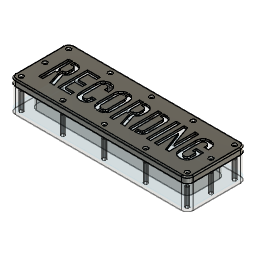
RECORDING sign (Autodesk Fusion 360 design; units mm, degrees)
Autodesk Fusion 360 part; units mm, degrees
note: some values were not read from the file. Set by a fixed rule: which sketch regions a step uses.
(part 1 of 2)
sketch "Esquisse1" plane through (0, 0, 0) normal (0, 0, 1) x (1, 0, 0)
  line L0 (0, 0) -> (300, 0)
  line L1 (300, 0) -> (300, -100)
  line L2 (300, -100) -> (0, -100)
  line L3 (0, -100) -> (0, 0)
  circle A0 centre (10, -10) radius 1.7
  circle A1 centre (290, -10) radius 1.7
  circle A2 centre (10, -90) radius 1.7
  circle A3 centre (290, -90) radius 1.7
  circle A4 centre (150, -10) radius 1.7
  circle A5 centre (150, -90) radius 1.7
  circle A6 centre (80, -10) radius 1.7
  circle A7 centre (80, -90) radius 1.7
  circle A8 centre (10, -50) radius 1.7
  circle A9 centre (290, -50) radius 1.7
  circle A10 centre (220, -10) radius 1.7
  circle A11 centre (220, -90) radius 1.7
  line L4 (27.716637, -53.851447) -> (27.716637, -47.661624)
  line L5 (27.716637, -47.661624) -> (36.932595, -47.661624)
  spline S0 degree 2 poles (36.932595, -47.661624) (39.580462, -47.661624) (41.041949, -46.200137) knots 0 0 0 1 1 1
  spline S1 degree 2 poles (41.041949, -46.200137) (42.503434, -44.73865) (42.503434, -42.125173) knots 0 0 0 1 1 1
  line L6 (42.503434, -42.125173) -> (42.503434, -37.035763)
  spline S2 degree 2 poles (42.503434, -37.035763) (42.503434, -34.250345) (41.041949, -32.702889) knots 0 0 0 1 1 1
  spline S3 degree 2 poles (41.041949, -32.702889) (39.580462, -31.155434) (36.932595, -31.155434) knots 0 0 0 1 1 1
  line L7 (36.932595, -31.155434) -> (27.716637, -31.155434)
  line L8 (27.716637, -31.155434) -> (27.716637, -24.965611)
  line L9 (27.716637, -24.965611) -> (36.348, -24.965611)
  spline S4 degree 2 poles (36.348, -24.965611) (40.371383, -24.965611) (43.208385, -26.289544) knots 0 0 0 1 1 1
  spline S5 degree 2 poles (43.208385, -26.289544) (46.045387, -27.613478) (47.541261, -30.158181) knots 0 0 0 1 1 1
  spline S6 degree 2 poles (47.541261, -30.158181) (49.037133, -32.702889) (49.037133, -36.313617) knots 0 0 0 1 1 1
  line L10 (49.037133, -36.313617) -> (49.037133, -42.159562)
  spline S7 degree 2 poles (49.037133, -42.159562) (49.037133, -45.873451) (47.541261, -48.486934) knots 0 0 0 1 1 1
  spline S8 degree 2 poles (47.541261, -48.486934) (46.045387, -51.100411) (43.208385, -52.475924) knots 0 0 0 1 1 1
  spline S9 degree 2 poles (43.208385, -52.475924) (40.371383, -53.851447) (36.348, -53.851447) knots 0 0 0 1 1 1
  line L11 (36.348, -53.851447) -> (27.716637, -53.851447)
  line L12 (24.656115, -75) -> (24.656115, -24.965611)
  line L13 (24.656115, -24.965611) -> (31.189815, -24.965611)
  line L14 (31.189815, -24.965611) -> (31.189815, -75)
  line L15 (31.189815, -75) -> (24.656115, -75)
  line L16 (43.294354, -75) -> (36.313612, -52.303987)
  line L17 (36.313612, -52.303987) -> (42.469044, -50.722146)
  line L18 (42.469044, -50.722146) -> (50.447038, -75)
  line L19 (50.447038, -75) -> (43.294354, -75)
  line L20 (56.464918, -75) -> (56.464918, -25)
  line L21 (56.464918, -25) -> (62.998617, -25)
  line L22 (62.998617, -25) -> (62.998617, -75)
  line L23 (62.998617, -75) -> (56.464918, -75)
  line L24 (59.869321, -75) -> (59.869321, -68.810177)
  line L25 (59.869321, -68.810177) -> (77.922962, -68.810177)
  line L26 (77.922962, -68.810177) -> (77.922962, -75)
  line L27 (77.922962, -75) -> (59.869321, -75)
  line L28 (59.869321, -53.26685) -> (59.869321, -47.077031)
  line L29 (59.869321, -47.077031) -> (76.203568, -47.077031)
  line L30 (76.203568, -47.077031) -> (76.203568, -53.26685)
  line L31 (76.203568, -53.26685) -> (59.869321, -53.26685)
  line L32 (59.869321, -31.189818) -> (59.869321, -25)
  line L33 (59.869321, -25) -> (77.922962, -25)
  line L34 (77.922962, -25) -> (77.922962, -31.189818)
  line L35 (77.922962, -31.189818) -> (59.869321, -31.189818)
  spline S10 degree 2 poles (94.704254, -75.515819) (91.02475, -75.515819) (88.428467, -74.002752) knots 0 0 0 1 1 1
  spline S11 degree 2 poles (88.428467, -74.002752) (85.832179, -72.489686) (84.456666, -69.635487) knots 0 0 0 1 1 1
  spline S12 degree 2 poles (84.456666, -69.635487) (83.081148, -66.781292) (83.081148, -62.723522) knots 0 0 0 1 1 1
  line L36 (83.081148, -62.723522) -> (83.081148, -37.310865)
  spline S13 degree 2 poles (83.081148, -37.310865) (83.081148, -33.218708) (84.456666, -30.364509) knots 0 0 0 1 1 1
  spline S14 degree 2 poles (84.456666, -30.364509) (85.832179, -27.510314) (88.428467, -25.997248) knots 0 0 0 1 1 1
  spline S15 degree 2 poles (88.428467, -25.997248) (91.02475, -24.484181) (94.704254, -24.484181) knots 0 0 0 1 1 1
  spline S16 degree 2 poles (94.704254, -24.484181) (98.418148, -24.484181) (101.014431, -25.997248) knots 0 0 0 1 1 1
  spline S17 degree 2 poles (101.014431, -25.997248) (103.610723, -27.510314) (104.969042, -30.364509) knots 0 0 0 1 1 1
  spline S18 degree 2 poles (104.969042, -30.364509) (106.32736, -33.218708) (106.32736, -37.276478) knots 0 0 0 1 1 1
  line L37 (106.32736, -37.276478) -> (106.32736, -39.408526)
  line L38 (106.32736, -39.408526) -> (99.724891, -39.408526)
  line L39 (99.724891, -39.408526) -> (99.724891, -37.276478)
  spline S19 degree 2 poles (99.724891, -37.276478) (99.724891, -35.213203) (99.140289, -33.786106) knots 0 0 0 1 1 1
  spline S20 degree 2 poles (99.140289, -33.786106) (98.555706, -32.359009) (97.438095, -31.602473) knots 0 0 0 1 1 1
  spline S21 degree 2 poles (97.438095, -31.602473) (96.320489, -30.845942) (94.704254, -30.845942) knots 0 0 0 1 1 1
  spline S22 degree 2 poles (94.704254, -30.845942) (92.331493, -30.845942) (91.00756, -32.530947) knots 0 0 0 1 1 1
  spline S23 degree 2 poles (91.00756, -32.530947) (89.683626, -34.215956) (89.683626, -37.310865) knots 0 0 0 1 1 1
  line L40 (89.683626, -37.310865) -> (89.683626, -62.723522)
  spline S24 degree 2 poles (89.683626, -62.723522) (89.683626, -65.784044) (91.00756, -67.469049) knots 0 0 0 1 1 1
  spline S25 degree 2 poles (91.00756, -67.469049) (92.331493, -69.154058) (94.704254, -69.154058) knots 0 0 0 1 1 1
  spline S26 degree 2 poles (94.704254, -69.154058) (97.111404, -69.154058) (98.418148, -67.469049) knots 0 0 0 1 1 1
  spline S27 degree 2 poles (98.418148, -67.469049) (99.724891, -65.784044) (99.724891, -62.723522) knots 0 0 0 1 1 1
  line L41 (99.724891, -62.723522) -> (99.724891, -60.591474)
  line L42 (99.724891, -60.591474) -> (106.32736, -60.591474)
  line L43 (106.32736, -60.591474) -> (106.32736, -62.723522)
  spline S28 degree 2 poles (106.32736, -62.723522) (106.32736, -66.781292) (104.969042, -69.635487) knots 0 0 0 1 1 1
  spline S29 degree 2 poles (104.969042, -69.635487) (103.610723, -72.489686) (101.014431, -74.002752) knots 0 0 0 1 1 1
  spline S30 degree 2 poles (101.014431, -74.002752) (98.418148, -75.515819) (94.704254, -75.515819) knots 0 0 0 1 1 1
  spline S31 degree 2 poles (124.931219, -75.515819) (121.010998, -75.515819) (118.225572, -74.037137) knots 0 0 0 1 1 1
  spline S32 degree 2 poles (118.225572, -74.037137) (115.440157, -72.55846) (113.97867, -69.755845) knots 0 0 0 1 1 1
  spline S33 degree 2 poles (113.97867, -69.755845) (112.517183, -66.953235) (112.517183, -62.964234) knots 0 0 0 1 1 1
  line L44 (112.517183, -62.964234) -> (112.517183, -37.035763)
  spline S34 degree 2 poles (112.517183, -37.035763) (112.517183, -33.012381) (113.97867, -30.209765) knots 0 0 0 1 1 1
  spline S35 degree 2 poles (113.97867, -30.209765) (115.440157, -27.40715) (118.225572, -25.945668) knots 0 0 0 1 1 1
  spline S36 degree 2 poles (118.225572, -25.945668) (121.010998, -24.484181) (124.931219, -24.484181) knots 0 0 0 1 1 1
  spline S37 degree 2 poles (124.931219, -24.484181) (128.88582, -24.484181) (131.654051, -25.945668) knots 0 0 0 1 1 1
  spline S38 degree 2 poles (131.654051, -25.945668) (134.422272, -27.40715) (135.883758, -30.209765) knots 0 0 0 1 1 1
  spline S39 degree 2 poles (135.883758, -30.209765) (137.345245, -33.012381) (137.345245, -37.035763) knots 0 0 0 1 1 1
  line L45 (137.345245, -37.035763) -> (137.345245, -62.964234)
  spline S40 degree 2 poles (137.345245, -62.964234) (137.345245, -66.953235) (135.883758, -69.755845) knots 0 0 0 1 1 1
  spline S41 degree 2 poles (135.883758, -69.755845) (134.422272, -72.55846) (131.654051, -74.037137) knots 0 0 0 1 1 1
  spline S42 degree 2 poles (131.654051, -74.037137) (128.88582, -75.515819) (124.931219, -75.515819) knots 0 0 0 1 1 1
  spline S43 degree 2 poles (124.931219, -69.154058) (127.716635, -69.154058) (129.264086, -67.572217) knots 0 0 0 1 1 1
  spline S44 degree 2 poles (129.264086, -67.572217) (130.811546, -65.990372) (130.811546, -63.170562) knots 0 0 0 1 1 1
  line L46 (130.811546, -63.170562) -> (130.811546, -36.829436)
  spline S45 degree 2 poles (130.811546, -36.829436) (130.811546, -33.975239) (129.264086, -32.410588) knots 0 0 0 1 1 1
  spline S46 degree 2 poles (129.264086, -32.410588) (127.716635, -30.845942) (124.931219, -30.845942) knots 0 0 0 1 1 1
  spline S47 degree 2 poles (124.931219, -30.845942) (122.111404, -30.845942) (120.581148, -32.410588) knots 0 0 0 1 1 1
  spline S48 degree 2 poles (120.581148, -32.410588) (119.050882, -33.975239) (119.050882, -36.829436) knots 0 0 0 1 1 1
  line L47 (119.050882, -36.829436) -> (119.050882, -63.170562)
  spline S49 degree 2 poles (119.050882, -63.170562) (119.050882, -65.990372) (120.581148, -67.572217) knots 0 0 0 1 1 1
  spline S50 degree 2 poles (120.581148, -67.572217) (122.111404, -69.154058) (124.931219, -69.154058) knots 0 0 0 1 1 1
  line L48 (147.283352, -53.851447) -> (147.283352, -47.661624)
  line L49 (147.283352, -47.661624) -> (156.499307, -47.661624)
  spline S51 degree 2 poles (156.499307, -47.661624) (159.147175, -47.661624) (160.608661, -46.200137) knots 0 0 0 1 1 1
  spline S52 degree 2 poles (160.608661, -46.200137) (162.070148, -44.73865) (162.070148, -42.125173) knots 0 0 0 1 1 1
  line L50 (162.070148, -42.125173) -> (162.070148, -37.035763)
  spline S53 degree 2 poles (162.070148, -37.035763) (162.070148, -34.250345) (160.608661, -32.702889) knots 0 0 0 1 1 1
  spline S54 degree 2 poles (160.608661, -32.702889) (159.147175, -31.155434) (156.499307, -31.155434) knots 0 0 0 1 1 1
  line L51 (156.499307, -31.155434) -> (147.283352, -31.155434)
  line L52 (147.283352, -31.155434) -> (147.283352, -24.965611)
  line L53 (147.283352, -24.965611) -> (155.914715, -24.965611)
  spline S55 degree 2 poles (155.914715, -24.965611) (159.938095, -24.965611) (162.775095, -26.289544) knots 0 0 0 1 1 1
  spline S56 degree 2 poles (162.775095, -26.289544) (165.612104, -27.613478) (167.107981, -30.158181) knots 0 0 0 1 1 1
  spline S57 degree 2 poles (167.107981, -30.158181) (168.603847, -32.702889) (168.603847, -36.313617) knots 0 0 0 1 1 1
  line L54 (168.603847, -36.313617) -> (168.603847, -42.159562)
  spline S58 degree 2 poles (168.603847, -42.159562) (168.603847, -45.873451) (167.107981, -48.486934) knots 0 0 0 1 1 1
  spline S59 degree 2 poles (167.107981, -48.486934) (165.612104, -51.100411) (162.775095, -52.475924) knots 0 0 0 1 1 1
  spline S60 degree 2 poles (162.775095, -52.475924) (159.938095, -53.851447) (155.914715, -53.851447) knots 0 0 0 1 1 1
  line L55 (155.914715, -53.851447) -> (147.283352, -53.851447)
  line L56 (144.22283, -75) -> (144.22283, -24.965611)
  line L57 (144.22283, -24.965611) -> (150.756529, -24.965611)
  line L58 (150.756529, -24.965611) -> (150.756529, -75)
  line L59 (150.756529, -75) -> (144.22283, -75)
  line L60 (162.861069, -75) -> (155.880325, -52.303987)
  line L61 (155.880325, -52.303987) -> (162.035759, -50.722146)
  line L62 (162.035759, -50.722146) -> (170.01375, -75)
  line L63 (170.01375, -75) -> (162.861069, -75)
  line L64 (180.192573, -75) -> (180.192573, -68.810177)
  line L65 (180.192573, -68.810177) -> (189.305351, -68.810177)
  spline S61 degree 2 poles (189.305351, -68.810177) (191.093529, -68.810177) (192.056396, -67.72696) knots 0 0 0 1 1 1
  spline S62 degree 2 poles (192.056396, -67.72696) (193.019264, -66.643739) (193.019264, -64.718018) knots 0 0 0 1 1 1
  line L66 (193.019264, -64.718018) -> (193.019264, -35.28198)
  spline S63 degree 2 poles (193.019264, -35.28198) (193.019264, -33.356256) (192.056396, -32.27304) knots 0 0 0 1 1 1
  spline S64 degree 2 poles (192.056396, -32.27304) (191.093529, -31.189818) (189.305351, -31.189818) knots 0 0 0 1 1 1
  line L67 (189.305351, -31.189818) -> (180.192573, -31.189818)
  line L68 (180.192573, -31.189818) -> (180.192573, -25)
  line L69 (180.192573, -25) -> (189.099052, -25)
  spline S65 degree 2 poles (189.099052, -25) (194.119652, -25) (196.836326, -27.716641) knots 0 0 0 1 1 1
  spline S66 degree 2 poles (196.836326, -27.716641) (199.552963, -30.433288) (199.552963, -35.45392) knots 0 0 0 1 1 1
  line L70 (199.552963, -35.45392) -> (199.552963, -64.54608)
  spline S67 degree 2 poles (199.552963, -64.54608) (199.552963, -67.847319) (198.314979, -70.202889) knots 0 0 0 1 1 1
  spline S68 degree 2 poles (198.314979, -70.202889) (197.077034, -72.55846) (194.738663, -73.77923) knots 0 0 0 1 1 1
  spline S69 degree 2 poles (194.738663, -73.77923) (192.400291, -75) (189.064644, -75) knots 0 0 0 1 1 1
  line L71 (189.064644, -75) -> (180.192573, -75)
  line L72 (176.031635, -75) -> (176.031635, -25)
  line L73 (176.031635, -25) -> (182.565353, -25)
  line L74 (182.565353, -25) -> (182.565353, -75)
  line L75 (182.565353, -75) -> (176.031635, -75)
  line L76 (212.895477, -25) -> (212.895477, -75)
  line L77 (212.895477, -75) -> (206.361778, -75)
  line L78 (206.361778, -75) -> (206.361778, -25)
  line L79 (206.361778, -25) -> (212.895477, -25)
  line L80 (219.704254, -74.965611) -> (219.704254, -24.999995)
  line L81 (219.704254, -24.999995) -> (225.412643, -24.999995)
  line L82 (225.412643, -24.999995) -> (239.099052, -63.3425)
  line L83 (239.099052, -63.3425) -> (238.032997, -64.236588)
  line L84 (238.032997, -64.236588) -> (238.032997, -24.999995)
  line L85 (238.032997, -24.999995) -> (244.25721, -24.999995)
  line L86 (244.25721, -24.999995) -> (244.25721, -74.965611)
  line L87 (244.25721, -74.965611) -> (238.480041, -74.965611)
  line L88 (238.480041, -74.965611) -> (224.862449, -37.826684)
  line L89 (224.862449, -37.826684) -> (225.928467, -36.932597)
  line L90 (225.928467, -36.932597) -> (225.928467, -74.965611)
  line L91 (225.928467, -74.965611) -> (219.704254, -74.965611)
  line L92 (263.170593, -48.074279) -> (275.343902, -48.074279)
  line L93 (275.343902, -48.074279) -> (275.343902, -62.689133)
  spline S70 degree 2 poles (275.343902, -62.689133) (275.343902, -66.746907) (273.93399, -69.618297) knots 0 0 0 1 1 1
  spline S71 degree 2 poles (273.93399, -69.618297) (272.524078, -72.489686) (269.841812, -74.002752) knots 0 0 0 1 1 1
  spline S72 degree 2 poles (269.841812, -74.002752) (267.159584, -75.515819) (263.342521, -75.515819) knots 0 0 0 1 1 1
  spline S73 degree 2 poles (263.342521, -75.515819) (259.45668, -75.515819) (256.722839, -74.088721) knots 0 0 0 1 1 1
  spline S74 degree 2 poles (256.722839, -74.088721) (253.988998, -72.661624) (252.56192, -69.962173) knots 0 0 0 1 1 1
  spline S75 degree 2 poles (252.56192, -69.962173) (251.134804, -67.262721) (251.134804, -63.411279) knots 0 0 0 1 1 1
  line L94 (251.134804, -63.411279) -> (251.134804, -37.310865)
  spline S76 degree 2 poles (251.134804, -37.310865) (251.134804, -33.218708) (252.544716, -30.364509) knots 0 0 0 1 1 1
  spline S77 degree 2 poles (252.544716, -30.364509) (253.954628, -27.510314) (256.636894, -25.997248) knots 0 0 0 1 1 1
  spline S78 degree 2 poles (256.636894, -25.997248) (259.319122, -24.484181) (263.136185, -24.484181) knots 0 0 0 1 1 1
  spline S79 degree 2 poles (263.136185, -24.484181) (266.884468, -24.484181) (269.515159, -25.945668) knots 0 0 0 1 1 1
  spline S80 degree 2 poles (269.515159, -25.945668) (272.145813, -27.40715) (273.538521, -30.192571) knots 0 0 0 1 1 1
  spline S81 degree 2 poles (273.538521, -30.192571) (274.931228, -32.977991) (274.931228, -36.9326) knots 0 0 0 1 1 1
  line L95 (274.931228, -36.9326) -> (274.931228, -39.408526)
  line L96 (274.931228, -39.408526) -> (267.984894, -39.408526)
  line L97 (267.984894, -39.408526) -> (267.984894, -36.9326)
  spline S82 degree 2 poles (267.984894, -36.9326) (267.984894, -34.009628) (266.729706, -32.427783) knots 0 0 0 1 1 1
  spline S83 degree 2 poles (266.729706, -32.427783) (265.474556, -30.845942) (263.136185, -30.845942) knots 0 0 0 1 1 1
  spline S84 degree 2 poles (263.136185, -30.845942) (260.522697, -30.845942) (259.095619, -32.530947) knots 0 0 0 1 1 1
  spline S85 degree 2 poles (259.095619, -32.530947) (257.668503, -34.215956) (257.668503, -37.310865) knots 0 0 0 1 1 1
  line L98 (257.668503, -37.310865) -> (257.668503, -63.411279)
  spline S86 degree 2 poles (257.668503, -63.411279) (257.668503, -66.127925) (259.147194, -67.640991) knots 0 0 0 1 1 1
  spline S87 degree 2 poles (259.147194, -67.640991) (260.625885, -69.154058) (263.342521, -69.154058) knots 0 0 0 1 1 1
  spline S88 degree 2 poles (263.342521, -69.154058) (265.9216, -69.154058) (267.365883, -67.486243) knots 0 0 0 1 1 1
  spline S89 degree 2 poles (267.365883, -67.486243) (268.810203, -65.818434) (268.810203, -62.792296) knots 0 0 0 1 1 1
  line L99 (268.810203, -62.792296) -> (268.810203, -54.264102)
  line L100 (268.810203, -54.264102) -> (263.170593, -54.264102)
  line L101 (263.170593, -54.264102) -> (263.170593, -48.074279)
  line L102 (31.189815, -24.965611) -> (34.189815, -24.965611)
  line L103 (34.189815, -24.965611) -> (34.189815, -31.155434)
  line L104 (34.189815, -31.155434) -> (31.189815, -31.155434)
  line L105 (31.189815, -31.155434) -> (31.189815, -24.965611)
  line L106 (36.799999, -53.999999) -> (33.799999, -53.999999)
  line L107 (33.799999, -53.999999) -> (33.799999, -47.661624)
  line L108 (33.799999, -47.661624) -> (36.799999, -47.661624)
  line L109 (36.799999, -47.661624) -> (36.799999, -53.999999)
  line L110 (123.500002, -31.5) -> (126.500002, -31.5)
  line L111 (126.500002, -31.5) -> (126.500002, -24)
  line L112 (126.500002, -24) -> (123.500002, -24)
  line L113 (123.500002, -24) -> (123.500002, -31.5)
  line L114 (123.500002, -68.500001) -> (126.500002, -68.500001)
  line L115 (126.500002, -68.500001) -> (126.500002, -76.000001)
  line L116 (126.500002, -76.000001) -> (123.500002, -76.000001)
  line L117 (123.500002, -76.000001) -> (123.500002, -68.500001)
  line L118 (150.756529, -24.965611) -> (153.756529, -24.965611)
  line L119 (153.756529, -24.965611) -> (153.756529, -31.155434)
  line L120 (153.756529, -31.155434) -> (150.756529, -31.155434)
  line L121 (150.756529, -31.155434) -> (150.756529, -24.965611)
  line L122 (156.349997, -53.899999) -> (153.349997, -53.899999)
  line L123 (153.349997, -53.899999) -> (153.349997, -47.661624)
  line L124 (153.349997, -47.661624) -> (156.349997, -47.661624)
  line L125 (156.349997, -47.661624) -> (156.349997, -53.899999)
  line L126 (182.565353, -25) -> (185.565353, -25)
  line L127 (185.565353, -25) -> (185.565353, -31.189818)
  line L128 (185.565353, -31.189818) -> (182.565353, -31.189818)
  line L129 (182.565353, -31.189818) -> (182.565353, -25)
  line L130 (182.565353, -68.810177) -> (185.565353, -68.810177)
  line L131 (185.565353, -68.810177) -> (185.565353, -75.000001)
  line L132 (185.565353, -75.000001) -> (182.565353, -75.000001)
  line L133 (182.565353, -75.000001) -> (182.565353, -68.810177)
  dimension "d35" = 300
  dimension "d36" = 100
  dimension "d37" = 3.4
  dimension "d38" = 3.4
  dimension "d39" = 3.4
  dimension "d40" = 3.4
  dimension "d41" = 3.4
  dimension "d42" = 3.4
  dimension "d43" = 3.4
  dimension "d44" = 3.4
  dimension "d45" = 3.4
  dimension "d46" = 3.4
  dimension "d47" = 3.4
  dimension "d48" = 3.4
  dimension "d50" = 3
  dimension "d51" = 3
  dimension "d52" = 3
  dimension "d53" = 3
  dimension "d54" = 3
  dimension "d55" = 3
  constraint horizontal L0
  constraint vertical L1
  constraint horizontal L2
  constraint vertical L3
  constraint coincident L0.start L3.end
  constraint horizontal L102
  constraint vertical L103
  constraint horizontal L104
  constraint vertical L105
  constraint horizontal L106
  constraint vertical L107
  constraint horizontal L108
  constraint vertical L109
  constraint horizontal L110
  constraint vertical L111
  constraint horizontal L112
  constraint vertical L113
  constraint horizontal L114
  constraint vertical L115
  constraint horizontal L116
  constraint vertical L117
  constraint horizontal L118
  constraint vertical L119
  constraint horizontal L120
  constraint vertical L121
  constraint horizontal L122
  constraint vertical L123
  constraint horizontal L124
  constraint vertical L125
  constraint horizontal L126
  constraint vertical L127
  constraint horizontal L128
  constraint vertical L129
  constraint horizontal L130
  constraint vertical L131
  constraint horizontal L132
  constraint vertical L133
  measures "d35" distance of L0.start L0.end
  measures "d36" distance of L0.start L2.end
  measures "d37" diameter of A0
  measures "d38" diameter of A1
  measures "d39" diameter of A2
  measures "d40" diameter of A3
  measures "d41" diameter of A4
  measures "d42" diameter of A5
  measures "d43" diameter of A6
  measures "d44" diameter of A7
  measures "d45" diameter of A8
  measures "d46" diameter of A9
  measures "d47" diameter of A10
  measures "d48" diameter of A11
extrude "Extrusion5" add sketch "Esquisse1" along normal blind 10 contours L0 L1 L2 L3 | L5 S0 S1 L6 S2 S3 L7 L14 L104 L108 | L5 S9 L11 L16 L17 L107 L108 L109 | S9 L11 L16 L106 L107 L109 | L7 L9 L14 L102 L103 L104 L105 | S9 L16 L17 L109 | S9 L16 L109 | S31 S42 L115 L116 L117 | S31 S42 S43 S50 L115 L117 | S43 S50 L114 L115 L117 | S43 S44 L46 S45 S46 S47 S48 L47 S49 S50 L110 L111 L113 L114 L115 L117 | S36 S37 S46 S47 L111 L113 | S46 S47 L110 L111 L113 | S36 S37 L111 L112 L113 | L49 S51 S52 L50 S53 S54 L51 L58 L120 L124 | L49 S60 L55 L60 L61 L123 L124 L125 | S60 L55 L122 L123 L125 | L51 L53 L58 L118 L119 L120 L121 | S60 L60 L125 | L60 L61 L125 | L65 L71 L74 L130 L131 L132 L133 | L65 S61 S62 L66 S63 S64 L67 L74 L128 L130 | L67 L69 L74 L126 L127 L128 L129 picked at (42.903127, -14.357499) picked at (36.831083, -38.617607) picked at (34.63787, -51.272353) picked at (35.649333, -53.950482) picked at (32.189815, -27.028885) picked at (36.633965, -52.776747) picked at (36.796095, -53.85988) picked at (124.977074, -75.838607) picked at (125.72501, -73.362581) picked at (124.977074, -68.71802) picked at (122.971103, -54.390186) picked at (125.72501, -26.637048) picked at (124.977074, -31.281981) picked at (124.977074, -24.161394) picked at (156.392224, -38.617607) picked at (154.193439, -51.272353) picked at (156.204903, -53.866267) picked at (151.756529, -27.028885) picked at (156.351664, -53.841872) picked at (156.193439, -52.772758) picked at (184.565353, -72.936726) picked at (186.04999, -45.093992) picked at (183.565353, -27.063273) makes body 1
chamfer "Chanfrein1" distance 2 angle 45 1 edges at (8.415044, -9.385254, 10) on bodies 1
chamfer "Chanfrein2" distance 2 angle 45 11 edges at (78.415044, -9.385254, 10) (148.415044, -9.385254, 10) (218.415044, -9.385254, 10) (288.415044, -9.385254, 10) (288.415044, -49.385254, 10) (288.415044, -89.385254, 10) (218.415044, -89.385254, 10) (148.415044, -89.385254, 10) (78.415044, -89.385254, 10) (8.415044, -89.385254, 10) (8.415044, -49.385254, 10) on bodies 1
fillet "Congé1" radius 10 4 edges at (300, 0, 5) (300, -100, 5) (0, 0, 5) (0, -100, 5) on bodies 1
fillet "Congé2" radius 2 8 edges at (2.928932, -97.071068, 10) (150, -100, 10) (297.071068, -97.071068, 10) (300, -50, 10) (297.071068, -2.928932, 10) (150, 0, 10) (2.928932, -2.928932, 10) (0, -50, 10) on bodies 1
sketch "Esquisse2" plane through (0, 0, 0) normal (0, 0, -1) x (1, 0, 0)
  arc A0 (10, 100) -> (0, 90) centre (10, 90) ccw
  line L0 (0, 90) -> (0, 10)
  arc A1 (0, 10) -> (10, 0) centre (10, 10) ccw
  line L1 (10, 0) -> (290, 0)
  arc A2 (290, 0) -> (300, 10) centre (290, 10) ccw
  line L2 (300, 10) -> (300, 90)
  arc A3 (300, 90) -> (290, 100) centre (290, 90) ccw
  line L3 (290, 100) -> (10, 100)
  circle A4 centre (290, 50) radius 1.7
  circle A5 centre (220, 10) radius 1.7
  line L4 (77.922962, 31.189818) -> (77.922962, 25)
  line L5 (77.922962, 25) -> (56.464918, 25)
  line L6 (56.464918, 25) -> (56.464918, 75)
  line L7 (56.464918, 75) -> (77.922962, 75)
  line L8 (77.922962, 75) -> (77.922962, 68.810177)
  line L9 (77.922962, 68.810177) -> (62.998617, 68.810177)
  line L10 (62.998617, 68.810177) -> (62.998617, 53.26685)
  line L11 (62.998617, 53.26685) -> (76.203568, 53.26685)
  line L12 (76.203568, 53.26685) -> (76.203568, 47.077031)
  line L13 (76.203568, 47.077031) -> (62.998617, 47.077031)
  line L14 (62.998617, 47.077031) -> (62.998617, 31.189818)
  line L15 (62.998617, 31.189818) -> (77.922962, 31.189818)
  circle A6 centre (80, 10) radius 1.7
  circle A7 centre (290, 90) radius 1.7
  circle A8 centre (150, 10) radius 1.7
  circle A9 centre (10, 90) radius 1.7
  circle A10 centre (220, 90) radius 1.7
  circle A11 centre (150, 90) radius 1.7
  circle A12 centre (10, 10) radius 1.7
  circle A13 centre (10, 50) radius 1.7
  circle A14 centre (290, 10) radius 1.7
  line L16 (123.500002, 75.463757) -> (123.500002, 69.038304)
  spline S0 degree 2 poles (120.581148, 67.572217) (121.697453, 68.726152) (123.500002, 69.038304) knots 0 0 0 0.72948894 0.72948894 0.72948894
  spline S1 degree 2 poles (119.050882, 63.170562) (119.050882, 65.990372) (120.581148, 67.572217) knots 0 0 0 1 1 1
  line L17 (119.050882, 63.170562) -> (119.050882, 36.829436)
  spline S2 degree 2 poles (120.581148, 32.410588) (119.050882, 33.975239) (119.050882, 36.829436) knots 0 0 0 1 1 1
  spline S3 degree 2 poles (123.500002, 30.960437) (121.697453, 31.269196) (120.581148, 32.410588) knots 0.27051106 0.27051106 0.27051106 1 1 1
  line L18 (123.500002, 30.960437) -> (123.500002, 24.535638)
  spline S4 degree 2 poles (118.225572, 25.945668) (120.488344, 24.758413) (123.500002, 24.535638) knots 0 0 0 0.81236119 0.81236119 0.81236119
  spline S5 degree 2 poles (113.97867, 30.209765) (115.440157, 27.40715) (118.225572, 25.945668) knots 0 0 0 1 1 1
  spline S6 degree 2 poles (112.517183, 37.035763) (112.517183, 33.012381) (113.97867, 30.209765) knots 0 0 0 1 1 1
  line L19 (112.517183, 37.035763) -> (112.517183, 62.964234)
  spline S7 degree 2 poles (113.97867, 69.755845) (112.517183, 66.953235) (112.517183, 62.964234) knots 0 0 0 1 1 1
  spline S8 degree 2 poles (118.225572, 74.037137) (115.440157, 72.55846) (113.97867, 69.755845) knots 0 0 0 1 1 1
  spline S9 degree 2 poles (123.500002, 75.463757) (120.488344, 75.238361) (118.225572, 74.037137) knots 0.18763881 0.18763881 0.18763881 1 1 1
  line L20 (31.189815, 47.661624) -> (31.189815, 24.965611)
  line L21 (31.189815, 24.965611) -> (24.656115, 24.965611)
  line L22 (24.656115, 24.965611) -> (24.656115, 75)
  line L23 (24.656115, 75) -> (31.189815, 75)
  line L24 (31.189815, 75) -> (31.189815, 53.851447)
  line L25 (31.189815, 53.851447) -> (33.799999, 53.851447)
  line L26 (33.799999, 53.851447) -> (33.799999, 47.661624)
  line L27 (33.799999, 47.661624) -> (31.189815, 47.661624)
  line L28 (36.932595, 47.661624) -> (36.799999, 47.661624)
  line L29 (36.799999, 47.661624) -> (36.799999, 53.885346)
  line L30 (36.799999, 53.885346) -> (43.294354, 75)
  line L31 (43.294354, 75) -> (50.447038, 75)
  line L32 (50.447038, 75) -> (43.067424, 52.543078)
  spline S10 degree 2 poles (43.208385, 52.475924) (43.138267, 52.509921) (43.067424, 52.543078) knots 0 0 0 0.02471554 0.02471554 0.02471554
  spline S11 degree 2 poles (47.541261, 48.486934) (46.045387, 51.100411) (43.208385, 52.475924) knots 0 0 0 1 1 1
  spline S12 degree 2 poles (49.037133, 42.159562) (49.037133, 45.873451) (47.541261, 48.486934) knots 0 0 0 1 1 1
  line L33 (49.037133, 42.159562) -> (49.037133, 36.313617)
  spline S13 degree 2 poles (47.541261, 30.158181) (49.037133, 32.702889) (49.037133, 36.313617) knots 0 0 0 1 1 1
  spline S14 degree 2 poles (43.208385, 26.289544) (46.045387, 27.613478) (47.541261, 30.158181) knots 0 0 0 1 1 1
  spline S15 degree 2 poles (36.348, 24.965611) (40.371383, 24.965611) (43.208385, 26.289544) knots 0 0 0 1 1 1
  line L34 (36.348, 24.965611) -> (34.189815, 24.965611)
  line L35 (34.189815, 24.965611) -> (34.189815, 31.155434)
  line L36 (34.189815, 31.155434) -> (36.932595, 31.155434)
  spline S16 degree 2 poles (41.041949, 32.702889) (39.580462, 31.155434) (36.932595, 31.155434) knots 0 0 0 1 1 1
  spline S17 degree 2 poles (42.503434, 37.035763) (42.503434, 34.250345) (41.041949, 32.702889) knots 0 0 0 1 1 1
  line L37 (42.503434, 37.035763) -> (42.503434, 42.125173)
  spline S18 degree 2 poles (41.041949, 46.200137) (42.503434, 44.73865) (42.503434, 42.125173) knots 0 0 0 1 1 1
  spline S19 degree 2 poles (36.932595, 47.661624) (39.580462, 47.661624) (41.041949, 46.200137) knots 0 0 0 1 1 1
  circle A15 centre (80, 90) radius 1.7
  line L38 (126.500002, 69.009926) -> (126.500002, 75.453901)
  spline S20 degree 2 poles (131.654051, 74.037137) (129.452283, 75.213236) (126.500002, 75.453901) knots 0 0 0 0.79536996 0.79536996 0.79536996
  spline S21 degree 2 poles (135.883758, 69.755845) (134.422272, 72.55846) (131.654051, 74.037137) knots 0 0 0 1 1 1
  spline S22 degree 2 poles (137.345245, 62.964234) (137.345245, 66.953235) (135.883758, 69.755845) knots 0 0 0 1 1 1
  line L39 (137.345245, 62.964234) -> (137.345245, 37.035763)
  spline S23 degree 2 poles (135.883758, 30.209765) (137.345245, 33.012381) (137.345245, 37.035763) knots 0 0 0 1 1 1
  spline S24 degree 2 poles (131.654051, 25.945668) (134.422272, 27.40715) (135.883758, 30.209765) knots 0 0 0 1 1 1
  spline S25 degree 2 poles (126.500002, 24.545379) (129.452283, 24.783246) (131.654051, 25.945668) knots 0.20463004 0.20463004 0.20463004 1 1 1
  line L40 (126.500002, 24.545379) -> (126.500002, 30.988507)
  spline S26 degree 2 poles (129.264086, 32.410588) (128.18374, 31.318238) (126.500002, 30.988507) knots 0 0 0 0.69814529 0.69814529 0.69814529
  spline S27 degree 2 poles (130.811546, 36.829436) (130.811546, 33.975239) (129.264086, 32.410588) knots 0 0 0 1 1 1
  line L41 (130.811546, 36.829436) -> (130.811546, 63.170562)
  spline S28 degree 2 poles (129.264086, 67.572217) (130.811546, 65.990372) (130.811546, 63.170562) knots 0 0 0 1 1 1
  spline S29 degree 2 poles (126.500002, 69.009926) (128.18374, 68.676571) (129.264086, 67.572217) knots 0.30185471 0.30185471 0.30185471 1 1 1
  line L42 (156.499307, 47.661624) -> (156.349997, 47.661624)
  line L43 (156.349997, 47.661624) -> (156.349997, 53.830997)
  line L44 (156.349997, 53.830997) -> (162.861069, 75)
  line L45 (162.861069, 75) -> (170.01375, 75)
  line L46 (170.01375, 75) -> (162.634138, 52.543076)
  spline S30 degree 2 poles (162.775095, 52.475924) (162.704979, 52.50992) (162.634138, 52.543076) knots 0 0 0 0.02471486 0.02471486 0.02471486
  spline S31 degree 2 poles (167.107981, 48.486934) (165.612104, 51.100411) (162.775095, 52.475924) knots 0 0 0 1 1 1
  spline S32 degree 2 poles (168.603847, 42.159562) (168.603847, 45.873451) (167.107981, 48.486934) knots 0 0 0 1 1 1
  line L47 (168.603847, 42.159562) -> (168.603847, 36.313617)
  spline S33 degree 2 poles (167.107981, 30.158181) (168.603847, 32.702889) (168.603847, 36.313617) knots 0 0 0 1 1 1
  spline S34 degree 2 poles (162.775095, 26.289544) (165.612104, 27.613478) (167.107981, 30.158181) knots 0 0 0 1 1 1
  spline S35 degree 2 poles (155.914715, 24.965611) (159.938095, 24.965611) (162.775095, 26.289544) knots 0 0 0 1 1 1
  line L48 (155.914715, 24.965611) -> (153.756529, 24.965611)
  line L49 (153.756529, 24.965611) -> (153.756529, 31.155434)
  line L50 (153.756529, 31.155434) -> (156.499307, 31.155434)
  spline S36 degree 2 poles (160.608661, 32.702889) (159.147175, 31.155434) (156.499307, 31.155434) knots 0 0 0 1 1 1
  spline S37 degree 2 poles (162.070148, 37.035763) (162.070148, 34.250345) (160.608661, 32.702889) knots 0 0 0 1 1 1
  line L51 (162.070148, 37.035763) -> (162.070148, 42.125173)
  spline S38 degree 2 poles (160.608661, 46.200137) (162.070148, 44.73865) (162.070148, 42.125173) knots 0 0 0 1 1 1
  spline S39 degree 2 poles (156.499307, 47.661624) (159.147175, 47.661624) (160.608661, 46.200137) knots 0 0 0 1 1 1
  spline S40 degree 2 poles (104.969042, 69.635487) (103.610723, 72.489686) (101.014431, 74.002752) knots 0 0 0 1 1 1
  spline S41 degree 2 poles (106.32736, 62.723522) (106.32736, 66.781292) (104.969042, 69.635487) knots 0 0 0 1 1 1
  line L52 (106.32736, 62.723522) -> (106.32736, 60.591474)
  line L53 (106.32736, 60.591474) -> (99.724891, 60.591474)
  line L54 (99.724891, 60.591474) -> (99.724891, 62.723522)
  spline S42 degree 2 poles (98.418148, 67.469049) (99.724891, 65.784044) (99.724891, 62.723522) knots 0 0 0 1 1 1
  spline S43 degree 2 poles (94.704254, 69.154058) (97.111404, 69.154058) (98.418148, 67.469049) knots 0 0 0 1 1 1
  spline S44 degree 2 poles (91.00756, 67.469049) (92.331493, 69.154058) (94.704254, 69.154058) knots 0 0 0 1 1 1
  spline S45 degree 2 poles (89.683626, 62.723522) (89.683626, 65.784044) (91.00756, 67.469049) knots 0 0 0 1 1 1
  line L55 (89.683626, 62.723522) -> (89.683626, 37.310865)
  spline S46 degree 2 poles (91.00756, 32.530947) (89.683626, 34.215956) (89.683626, 37.310865) knots 0 0 0 1 1 1
  spline S47 degree 2 poles (94.704254, 30.845942) (92.331493, 30.845942) (91.00756, 32.530947) knots 0 0 0 1 1 1
  spline S48 degree 2 poles (97.438095, 31.602473) (96.320489, 30.845942) (94.704254, 30.845942) knots 0 0 0 1 1 1
  spline S49 degree 2 poles (99.140289, 33.786106) (98.555706, 32.359009) (97.438095, 31.602473) knots 0 0 0 1 1 1
  spline S50 degree 2 poles (99.724891, 37.276478) (99.724891, 35.213203) (99.140289, 33.786106) knots 0 0 0 1 1 1
  line L56 (99.724891, 37.276478) -> (99.724891, 39.408526)
  line L57 (99.724891, 39.408526) -> (106.32736, 39.408526)
  line L58 (106.32736, 39.408526) -> (106.32736, 37.276478)
  spline S51 degree 2 poles (104.969042, 30.364509) (106.32736, 33.218708) (106.32736, 37.276478) knots 0 0 0 1 1 1
  spline S52 degree 2 poles (101.014431, 25.997248) (103.610723, 27.510314) (104.969042, 30.364509) knots 0 0 0 1 1 1
  spline S53 degree 2 poles (94.704254, 24.484181) (98.418148, 24.484181) (101.014431, 25.997248) knots 0 0 0 1 1 1
  spline S54 degree 2 poles (88.428467, 25.997248) (91.02475, 24.484181) (94.704254, 24.484181) knots 0 0 0 1 1 1
  spline S55 degree 2 poles (84.456666, 30.364509) (85.832179, 27.510314) (88.428467, 25.997248) knots 0 0 0 1 1 1
  spline S56 degree 2 poles (83.081148, 37.310865) (83.081148, 33.218708) (84.456666, 30.364509) knots 0 0 0 1 1 1
  line L59 (83.081148, 37.310865) -> (83.081148, 62.723522)
  spline S57 degree 2 poles (84.456666, 69.635487) (83.081148, 66.781292) (83.081148, 62.723522) knots 0 0 0 1 1 1
  spline S58 degree 2 poles (88.428467, 74.002752) (85.832179, 72.489686) (84.456666, 69.635487) knots 0 0 0 1 1 1
  spline S59 degree 2 poles (94.704254, 75.515819) (91.02475, 75.515819) (88.428467, 74.002752) knots 0 0 0 1 1 1
  spline S60 degree 2 poles (101.014431, 74.002752) (98.418148, 75.515819) (94.704254, 75.515819) knots 0 0 0 1 1 1
  line L60 (176.031635, 75) -> (182.565353, 75.000001)
  line L61 (182.565353, 75.000001) -> (182.565353, 25)
  line L62 (182.565353, 25) -> (176.031635, 25)
  line L63 (176.031635, 25) -> (176.031635, 75)
  line L64 (189.305351, 68.810177) -> (185.565353, 68.810177)
  line L65 (185.565353, 68.810177) -> (185.565353, 75.000001)
  line L66 (185.565353, 75.000001) -> (189.064644, 75)
  spline S61 degree 2 poles (194.738663, 73.77923) (192.400291, 75) (189.064644, 75) knots 0 0 0 1 1 1
  spline S62 degree 2 poles (198.314979, 70.202889) (197.077034, 72.55846) (194.738663, 73.77923) knots 0 0 0 1 1 1
  spline S63 degree 2 poles (199.552963, 64.54608) (199.552963, 67.847319) (198.314979, 70.202889) knots 0 0 0 1 1 1
  line L67 (199.552963, 64.54608) -> (199.552963, 35.45392)
  spline S64 degree 2 poles (196.836326, 27.716641) (199.552963, 30.433288) (199.552963, 35.45392) knots 0 0 0 1 1 1
  spline S65 degree 2 poles (189.099052, 25) (194.119652, 25) (196.836326, 27.716641) knots 0 0 0 1 1 1
  line L68 (189.099052, 25) -> (185.565353, 25)
  line L69 (185.565353, 25) -> (185.565353, 31.189818)
  line L70 (185.565353, 31.189818) -> (189.305351, 31.189818)
  spline S66 degree 2 poles (192.056396, 32.27304) (191.093529, 31.189818) (189.305351, 31.189818) knots 0 0 0 1 1 1
  spline S67 degree 2 poles (193.019264, 35.28198) (193.019264, 33.356256) (192.056396, 32.27304) knots 0 0 0 1 1 1
  line L71 (193.019264, 35.28198) -> (193.019264, 64.718018)
  spline S68 degree 2 poles (192.056396, 67.72696) (193.019264, 66.643739) (193.019264, 64.718018) knots 0 0 0 1 1 1
  spline S69 degree 2 poles (189.305351, 68.810177) (191.093529, 68.810177) (192.056396, 67.72696) knots 0 0 0 1 1 1
  line L72 (150.756529, 47.661624) -> (150.756529, 24.965611)
  line L73 (150.756529, 24.965611) -> (144.22283, 24.965611)
  line L74 (144.22283, 24.965611) -> (144.22283, 75)
  line L75 (144.22283, 75) -> (150.756529, 75)
  line L76 (150.756529, 75) -> (150.756529, 53.851447)
  line L77 (150.756529, 53.851447) -> (153.349997, 53.851447)
  line L78 (153.349997, 53.851447) -> (153.349997, 47.661624)
  line L79 (153.349997, 47.661624) -> (150.756529, 47.661624)
  line L80 (263.170593, 54.264102) -> (268.810203, 54.264102)
  line L81 (268.810203, 54.264102) -> (268.810203, 62.792296)
  spline S70 degree 2 poles (267.365883, 67.486243) (268.810203, 65.818434) (268.810203, 62.792296) knots 0 0 0 1 1 1
  spline S71 degree 2 poles (263.342521, 69.154058) (265.9216, 69.154058) (267.365883, 67.486243) knots 0 0 0 1 1 1
  spline S72 degree 2 poles (259.147194, 67.640991) (260.625885, 69.154058) (263.342521, 69.154058) knots 0 0 0 1 1 1
  spline S73 degree 2 poles (257.668503, 63.411279) (257.668503, 66.127925) (259.147194, 67.640991) knots 0 0 0 1 1 1
  line L82 (257.668503, 63.411279) -> (257.668503, 37.310865)
  spline S74 degree 2 poles (259.095619, 32.530947) (257.668503, 34.215956) (257.668503, 37.310865) knots 0 0 0 1 1 1
  spline S75 degree 2 poles (263.136185, 30.845942) (260.522697, 30.845942) (259.095619, 32.530947) knots 0 0 0 1 1 1
  spline S76 degree 2 poles (266.729706, 32.427783) (265.474556, 30.845942) (263.136185, 30.845942) knots 0 0 0 1 1 1
  spline S77 degree 2 poles (267.984894, 36.9326) (267.984894, 34.009628) (266.729706, 32.427783) knots 0 0 0 1 1 1
  line L83 (267.984894, 36.9326) -> (267.984894, 39.408526)
  line L84 (267.984894, 39.408526) -> (274.931228, 39.408526)
  line L85 (274.931228, 39.408526) -> (274.931228, 36.9326)
  spline S78 degree 2 poles (273.538521, 30.192571) (274.931228, 32.977991) (274.931228, 36.9326) knots 0 0 0 1 1 1
  spline S79 degree 2 poles (269.515159, 25.945668) (272.145813, 27.40715) (273.538521, 30.192571) knots 0 0 0 1 1 1
  spline S80 degree 2 poles (263.136185, 24.484181) (266.884468, 24.484181) (269.515159, 25.945668) knots 0 0 0 1 1 1
  spline S81 degree 2 poles (256.636894, 25.997248) (259.319122, 24.484181) (263.136185, 24.484181) knots 0 0 0 1 1 1
  spline S82 degree 2 poles (252.544716, 30.364509) (253.954628, 27.510314) (256.636894, 25.997248) knots 0 0 0 1 1 1
  spline S83 degree 2 poles (251.134804, 37.310865) (251.134804, 33.218708) (252.544716, 30.364509) knots 0 0 0 1 1 1
  line L86 (251.134804, 37.310865) -> (251.134804, 63.411279)
  spline S84 degree 2 poles (252.56192, 69.962173) (251.134804, 67.262721) (251.134804, 63.411279) knots 0 0 0 1 1 1
  spline S85 degree 2 poles (256.722839, 74.088721) (253.988998, 72.661624) (252.56192, 69.962173) knots 0 0 0 1 1 1
  spline S86 degree 2 poles (263.342521, 75.515819) (259.45668, 75.515819) (256.722839, 74.088721) knots 0 0 0 1 1 1
  spline S87 degree 2 poles (269.841812, 74.002752) (267.159584, 75.515819) (263.342521, 75.515819) knots 0 0 0 1 1 1
  spline S88 degree 2 poles (273.93399, 69.618297) (272.524078, 72.489686) (269.841812, 74.002752) knots 0 0 0 1 1 1
  spline S89 degree 2 poles (275.343902, 62.689133) (275.343902, 66.746907) (273.93399, 69.618297) knots 0 0 0 1 1 1
  line L87 (275.343902, 62.689133) -> (275.343902, 48.074279)
  line L88 (275.343902, 48.074279) -> (263.170593, 48.074279)
  line L89 (263.170593, 48.074279) -> (263.170593, 54.264102)
  line L90 (206.361778, 25) -> (206.361778, 75)
  line L91 (206.361778, 75) -> (212.895477, 75)
  line L92 (212.895477, 75) -> (212.895477, 25)
  line L93 (212.895477, 25) -> (206.361778, 25)
  line L94 (225.928467, 74.965611) -> (225.928467, 40.734006)
  line L95 (225.928467, 40.734006) -> (238.480041, 74.965611)
  line L96 (238.480041, 74.965611) -> (244.25721, 74.965611)
  line L97 (244.25721, 74.965611) -> (244.25721, 24.999995)
  line L98 (244.25721, 24.999995) -> (238.032997, 24.999995)
  line L99 (238.032997, 24.999995) -> (238.032997, 60.355944)
  line L100 (238.032997, 60.355944) -> (225.412643, 24.999995)
  line L101 (225.412643, 24.999995) -> (219.704254, 24.999995)
  line L102 (219.704254, 24.999995) -> (219.704254, 74.965611)
  line L103 (219.704254, 74.965611) -> (225.928467, 74.965611)
  line L104 (290, 100) -> (10, 100)
  arc A16 (10, 100) -> (0, 90) centre (10, 90) ccw
  line L105 (0, 90) -> (0, 10)
  arc A17 (0, 10) -> (10, 0) centre (10, 10) ccw
  line L106 (10, 0) -> (290, 0)
  arc A18 (290, 0) -> (300, 10) centre (290, 10) ccw
  line L107 (300, 10) -> (300, 90)
  arc A19 (300, 90) -> (290, 100) centre (290, 90) ccw
  line L108 (18, 82) -> (18, 18)
  line L109 (18, 18) -> (282, 18)
  line L110 (282, 18) -> (282, 82)
  line L111 (282, 82) -> (18, 82)
  dimension "d64" = -18
extrude "Extrusion6" cut sketch "Esquisse2" against normal blind 7 contours L108 L109 L110 L111 picked at (233.826212, 36.785311) bodies 1
sketch "Esquisse3" plane through (0, 0, 0) normal (0, 0, -1) x (1, 0, 0)
  line L0 (18, 18) -> (18, 82)
  line L1 (18, 82) -> (282, 82)
  line L2 (282, 82) -> (282, 18)
  line L3 (282, 18) -> (18, 18)
  arc A0 (10, 100) -> (0, 90) centre (10, 90) ccw
  line L4 (0, 90) -> (0, 10)
  arc A1 (0, 10) -> (10, 0) centre (10, 10) ccw
  line L5 (10, 0) -> (290, 0)
  arc A2 (290, 0) -> (300, 10) centre (290, 10) ccw
  line L6 (300, 10) -> (300, 90)
  arc A3 (300, 90) -> (290, 100) centre (290, 90) ccw
  line L7 (290, 100) -> (10, 100)
  circle A4 centre (290, 50) radius 1.7
  circle A5 centre (220, 10) radius 1.7
  circle A6 centre (80, 10) radius 1.7
  circle A7 centre (290, 90) radius 1.7
  circle A8 centre (150, 10) radius 1.7
  circle A9 centre (10, 90) radius 1.7
  circle A10 centre (220, 90) radius 1.7
  circle A11 centre (150, 90) radius 1.7
  circle A12 centre (10, 10) radius 1.7
  circle A13 centre (10, 50) radius 1.7
  circle A14 centre (290, 10) radius 1.7
  circle A15 centre (80, 90) radius 1.7
extrude "Extrusion1" add sketch "Esquisse3" along normal blind 35 separate body makes body 2 in component "Component"
fillet "Congé1'" radius 10 4 edges at (18, -82, -17.5) (18, -18, -17.5) (282, -18, -17.5) (282, -82, -17.5) on bodies 2 in component "Component"
sketch "Esquisse4" plane through (0, 0, -35) normal (0, 0, -1) x (1, 0, 0)
  circle A0 centre (290, 50) radius 1.7
  circle A1 centre (10, 10) radius 1.7
  circle A2 centre (80, 90) radius 1.7
  circle A3 centre (150, 10) radius 1.7
  circle A4 centre (220, 90) radius 1.7
  line L0 (282, 72) -> (282, 28)
  arc A5 (272, 18) -> (282, 28) centre (272, 28) ccw
  line L1 (272, 18) -> (28, 18)
  arc A6 (18, 28) -> (28, 18) centre (28, 28) ccw
  line L2 (18, 28) -> (18, 72)
  arc A7 (28, 82) -> (18, 72) centre (28, 72) ccw
  line L3 (28, 82) -> (272, 82)
  arc A8 (282, 72) -> (272, 82) centre (272, 72) ccw
  circle A9 centre (10, 50) radius 1.7
  circle A10 centre (80, 10) radius 1.7
  circle A11 centre (290, 90) radius 1.7
  circle A12 centre (220, 10) radius 1.7
  circle A13 centre (150, 90) radius 1.7
  circle A14 centre (10, 90) radius 1.7
  circle A15 centre (290, 10) radius 1.7
  line L4 (290, 100) -> (10, 100)
  arc A16 (10, 100) -> (0, 90) centre (10, 90) ccw
  line L5 (0, 90) -> (0, 10)
  arc A17 (0, 10) -> (10, 0) centre (10, 10) ccw
  line L6 (10, 0) -> (290, 0)
  arc A18 (290, 0) -> (300, 10) centre (290, 10) ccw
  line L7 (300, 10) -> (300, 90)
  arc A19 (300, 90) -> (290, 100) centre (290, 90) ccw